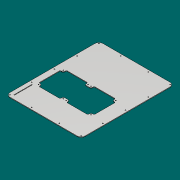
# Autodesk Inventor part: left_panel_amd
Saved by Autodesk Inventor 2018.2 (Build 222227000, 227)
## iProperties
Created: 2019-10-14
Part Number: left_panel_amd
Material: アルミニウム 6061
Document SubType Name: Modeling
Designer: gisen
Density: 2.7 g/cm^3
Appearance: アルミニウム - フラット
Author: gisen
Autodesk Inventor part; units mm, degrees
ref_plane "YZ Plane" through (0, 0, 0) normal (1, 0, 0) x (0, 1, 0)
ref_plane "XZ Plane" through (0, 0, 0) normal (0, 1, 0) x (-1, 0, 0)
ref_plane "XY Plane" through (0, 0, 0) normal (0, 0, 1) x (1, 0, 0)
sketch "スケッチ1" plane through (0, 0, 0) normal (0, 0, 1) x (1, 0, 0)
  line L0 (-170, -235) -> (170, -235)
  line L1 (190, -215) -> (190, 215)
  line L2 (170, 235) -> (-170, 235)
  line L3 (-190, 215) -> (-190, -215)
  line L4 (-190, -235) -> (190, 235) construction
  line L5 (190, -235) -> (-190, 235) construction
  circle A0 centre (-180, 225) radius 2.25
  circle A1 centre (180, 225) radius 2.25
  circle A2 centre (-180, -225) radius 2.25
  circle A3 centre (180, -225) radius 2.25
  arc A4 (-170, 235) -> (-190, 215) centre (-170, 215) ccw
  arc A5 (190, 215) -> (170, 235) centre (170, 215) ccw
  arc A6 (170, -235) -> (190, -215) centre (170, -215) ccw
  arc A7 (-190, -215) -> (-170, -235) centre (-170, -215) ccw
  point P0 (0, 0)
  dimension "d0" = 380
  dimension "d1" = 470
  dimension "d2" = 4.5
  dimension "d3" = 10
  dimension "d4" = 10
  dimension "d5" = 10
  dimension "d6" = 10
  dimension "d7" = 10
  dimension "d8" = 10
  dimension "d9" = 10
  dimension "d10" = 10
  dimension "d11" = 20
  constraints: 12 end point, 8 centre point, 8 point on circle, 8 point on line, 8 tangent, 6 equal radius, 2 midpoint, 2 parallel, 1 horizontal, 1 perpendicular
  measures "d0" distance of L5.end L4.end
  measures "d1" distance of L4.end L5.start
  measures "d2" diameter of A0
  measures "d3" distance from line of A0.centre L2
  measures "d4" distance from line of L3 A0.centre
  measures "d5" distance from line of A1.centre L2
  measures "d6" distance from line of L1 A1.centre
  measures "d7" distance from line of L1 A3.centre
  measures "d8" distance from line of L0 A3.centre
  measures "d9" distance from line of L0 A2.centre
  measures "d10" distance from line of L3 A2.centre
  measures "d11" radius of A4
extrude "押し出し1" add sketch "スケッチ1" along normal blind 3
sketch "スケッチ2" plane through (0, 0, 3) normal (0, 0, 1) x (1, 0, 0)
  circle A0 centre (-180, -225) radius 2.25 construction
  circle A1 centre (-180, -115) radius 2.25
  line L0 (-190, 215) -> (-190, -215) projected
  point P0 (0, 0)
  dimension "d14" = 110
  dimension "d15" = 10
  constraints: 1 centre point, 1 equal radius
  measures "d14" distance of A1.centre A0.centre
  measures "d15" distance from line of A1.centre L0
extrude "押し出し2" cut sketch "スケッチ2" against normal blind 10
sketch "スケッチ3" plane through (0, 0, 3) normal (0, 0, 1) x (1, 0, 0)
  line L0 (-167, -124.6) -> (-167, -215) construction
  line L1 (-170, -124.6) -> (-167, -124.6) construction
  line L2 (-170, -215) -> (-170, -124.6) construction
  line L3 (-170, -215) -> (-167, -215) construction
  line L4 (-170.2, -124.4) -> (-166.8, -124.4)
  line L5 (-166.8, -124.4) -> (-166.8, -215.2)
  line L6 (-166.8, -215.2) -> (-170.2, -215.2)
  line L7 (-170.2, -215.2) -> (-170.2, -124.4)
  point P0 (0, 0)
  dimension "d18" = 0.2
  constraints: 8 end point, 3 other
  measures "d18" distance between parallel lines of L2 L7
extrude "押し出し3" cut sketch "スケッチ3" against normal up to surface (3 mm away)
sketch "スケッチ4" plane through (0, 0, 3) normal (0, 0, 1) x (1, 0, 0)
  circle A0 centre (-180, -225) radius 2.25 construction
  circle A1 centre (-180, -115) radius 2.25 construction
  circle A2 centre (180, -225) radius 2.25 construction
  circle A3 centre (-180, 225) radius 2.25 construction
  circle A4 centre (180, 225) radius 2.25 construction
  circle A5 centre (-180, -225) radius 2.25 construction
  circle A6 centre (-180, -115) radius 2.25 construction
  circle A7 centre (-180, -225) radius 110 construction
  circle A8 centre (-180, 225) radius 2.25 construction
  circle A9 centre (-180, 225) radius 110 construction
  circle A10 centre (180, 225) radius 110 construction
  circle A11 centre (180, -225) radius 110 construction
  line L0 (-180, -225) -> (180, -225) construction
  line L1 (180, -225) -> (180, 225) construction
  line L2 (180, 225) -> (-180, 225) construction
  line L3 (-180, 225) -> (-180, -225) construction
  line L4 (-180, 0) -> (180, 0) construction
  circle A12 centre (-180, 115) radius 2.25
  circle A13 centre (-180, 0) radius 2.25
  circle A14 centre (-70, -225) radius 2.25
  circle A15 centre (70, -225) radius 2.25
  circle A16 centre (180, -115) radius 2.25
  circle A17 centre (180, 115) radius 2.25
  circle A18 centre (70, 225) radius 2.25
  circle A19 centre (-70, 225) radius 2.25
  circle A20 centre (180, 0) radius 2.25
  point P0 (0, 0)
  constraints: 13 centre point, 12 equal radius, 10 end point, 8 point on circle, 7 point on line, 6 coincident, 2 midpoint, 2 parallel, 1 horizontal, 1 perpendicular
extrude "押し出し4" cut sketch "スケッチ4" against normal up to surface (3 mm away)
sketch "スケッチ5" plane through (0, 0, 3) normal (0, 0, 1) x (1, 0, 0)
  line L0 (-160, -115) -> (-20, -115) construction
  line L1 (-20, -115) -> (-20, 25) construction
  line L2 (-20, 25) -> (-160, 25) construction
  line L3 (-160, 25) -> (-160, -115) construction
  line L4 (-20, -115) -> (120, -115) construction
  line L5 (120, -115) -> (120, 25) construction
  line L6 (120, 25) -> (-20, 25) construction
  line L7 (-20, 25) -> (-20, -115) construction
  line L8 (-170, -235) -> (170, -235) construction
  line L9 (-190, 215) -> (-190, -215) construction
  line L10 (-152.5, -107.5) -> (-27.5, -107.5) construction
  line L11 (-27.5, -107.5) -> (-27.5, 17.5) construction
  line L12 (-27.5, 17.5) -> (-152.5, 17.5) construction
  line L13 (-152.5, 17.5) -> (-152.5, -107.5) construction
  line L14 (-12.5, 17.5) -> (112.5, 17.5) construction
  line L15 (112.5, 17.5) -> (112.5, -107.5) construction
  line L16 (112.5, -107.5) -> (-12.5, -107.5) construction
  line L17 (-12.5, -107.5) -> (-12.5, 17.5) construction
  circle A0 centre (-152.5, 17.5) radius 2.25
  circle A1 centre (-27.5, 17.5) radius 2.25
  circle A2 centre (-152.5, -107.5) radius 2.25
  circle A3 centre (-27.5, -107.5) radius 2.25
  circle A4 centre (-12.5, -107.5) radius 2.25
  circle A5 centre (-12.5, 17.5) radius 2.25
  circle A6 centre (112.5, 17.5) radius 2.25
  circle A7 centre (112.5, -107.5) radius 2.25
  line L18 (-144, 25) -> (-144, 9)
  line L19 (-144, 9) -> (-160, 9)
  line L20 (-160, 9) -> (-160, -99)
  line L21 (-160, -99) -> (-144, -99)
  line L22 (-144, -99) -> (-144, -115)
  line L23 (-144, -115) -> (-36, -115)
  line L24 (-36, -115) -> (-36, -99)
  line L25 (-36, -99) -> (-4, -99)
  line L26 (-4, -99) -> (-4, -115)
  line L27 (-4, -115) -> (104, -115)
  line L28 (104, -115) -> (104, -99)
  line L29 (104, -99) -> (120, -99)
  line L30 (120, -99) -> (120, 9)
  line L31 (120, 9) -> (104, 9)
  line L32 (104, 9) -> (104, 25)
  line L33 (104, 25) -> (-4, 25)
  line L34 (-4, 25) -> (-4, 9)
  line L35 (-4, 9) -> (-36, 9)
  line L36 (-36, 9) -> (-36, 25)
  line L37 (-36, 25) -> (-144, 25)
  point P0 (0, 0)
  dimension "d23" = 140
  dimension "d24" = 0
  dimension "d25" = 120
  dimension "d26" = 30
  dimension "d27" = 125
  dimension "d28" = 125
  dimension "d29" = 7.5
  dimension "d30" = 7.5
  dimension "d31" = 7.5
  dimension "d32" = 7.5
  dimension "d33" = 7.5
  dimension "d34" = 4.5
  dimension "d35" = 16
  dimension "d36" = 16
  constraints: 72 end point, 20 perpendicular, 14 equal length, 13 point on line, 8 centre point, 8 coincident, 8 parallel, 7 equal radius, 4 horizontal, 1 vertical
  measures "d23" distance of L2.end L1.end
  measures "d24" distance between parallel lines of L1 L7
  measures "d25" distance between parallel lines of L8 L0
  measures "d26" distance between parallel lines of L9 L3
  measures "d27" distance of L12.end L11.end
  measures "d28" distance of L11.end L10.end
  measures "d29" distance between parallel lines of L12 L2
  measures "d30" distance between parallel lines of L0 L10
  measures "d31" distance between parallel lines of L3 L13
  measures "d32" distance between parallel lines of L4 L16
  measures "d33" distance between parallel lines of L5 L15
  measures "d34" diameter of A0
  measures "d35" distance between parallel lines of L19 L2
  measures "d36" distance between parallel lines of L3 L18
extrude "押し出し5" cut sketch "スケッチ5" against normal through all
fillet "フィレット1" radius 8 8 edges at (-144, 9, 1.5) (-144, -99, 1.5) (-36, -99, 1.5) (-4, -99, 1.5) (104, -99, 1.5) (104, 9, 1.5) (-4, 9, 1.5) (-36, 9, 1.5)
fillet "フィレット1" radius 5.3333 12 edges at (-144, 25, 1.5) (-160, 9, 1.5) (-160, -99, 1.5) (-144, -115, 1.5) (-36, -115, 1.5) (-4, -115, 1.5) (104, -115, 1.5) (120, -99, 1.5) (120, 9, 1.5) (104, 25, 1.5) (-4, 25, 1.5) (-36, 25, 1.5)
equation "\"d5\" = d3"
equation "\"d6\" = d4"
equation "\"d7\" = d6"
equation "\"d8\" = d5"
equation "\"d9\" = d8"
equation "\"d10\" = d7"
equation "\"d30\" = d29"
equation "\"d31\" = d30"
equation "\"d32\" = d30"
equation "\"d33\" = d31"
equation "\"d36\" = d35"
equation "\"d39\" = 0.5 * d35"
equation "\"d40\" = 0.333333 * d35"
